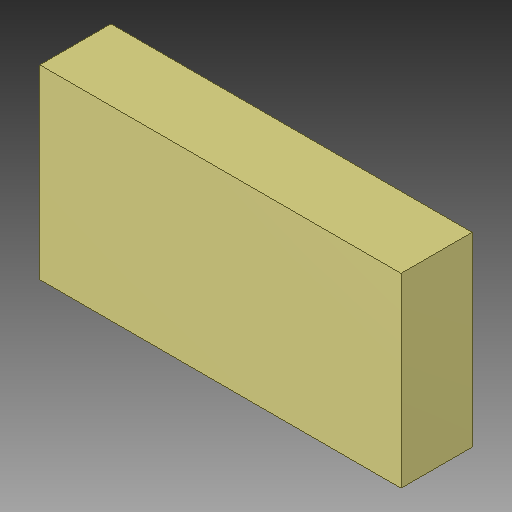
# Autodesk Inventor part: 1X02
Saved by Autodesk Inventor 2019 (Build 230136000, 136)
## iProperties
Created: 2019-10-02
Part Number: 1X02
Material: Generic
Document SubType Name: Modeling
Designer: rybit
Density: 1 g/cm^3
Appearance: 1X02, 1X02
Author: rybit
Autodesk Inventor part; units mm, degrees
ref_plane "YZ Plane" through (0, 0, 0) normal (1, 0, 0) x (0, 1, 0)
ref_plane "XZ Plane" through (0, 0, 0) normal (0, 1, 0) x (-1, 0, 0)
ref_plane "XY Plane" through (0, 0, 0) normal (0, 0, 1) x (1, 0, 0)
sketch "1X02, 1X02_8" plane through (0, 0, 0) normal (0, 0, 1) x (1, 0, 0)
  line L0 (-2.54, 1.3462) -> (2.54, 1.3462)
  line L1 (2.54, 1.3462) -> (2.54, -1.27)
  line L2 (2.54, -1.27) -> (-2.54, -1.27)
  line L3 (-2.54, -1.27) -> (-2.54, 1.3462)
  constraints: 8 end point
extrude "Extrusion1" add sketch "1X02, 1X02_8" along normal blind 1
body "Solid1"
